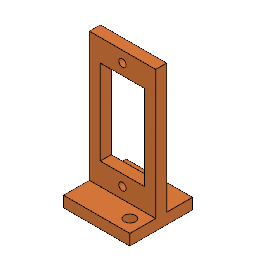
chassis laser 2x3mm (Autodesk Fusion 360 archive; units mm, degrees)
design "Version 3D vissée"
Autodesk Fusion 360 part; units mm, degrees
sketch "Sketch base" plane through (0, 0, 0) normal (0, 1, 0) x (1, 0, 0)
  line L0 (0, 0) -> (18, 0)
  line L1 (18, 0) -> (18, -3)
  line L2 (18, -3) -> (0, -3)
  line L3 (0, -3) -> (0, 0)
  dimension "d1" = 18
  dimension "d2" = 3
  constraint horizontal L0
  constraint vertical L1
  constraint horizontal L2
  constraint vertical L3
  constraint coincident L0.start L3.end
  measures "d1" distance of L0.start L0.end
  measures "d2" distance of L0.start L2.end
extrude "Extrude base" add sketch "Sketch base" along normal blind 38
sketch "Sketch face" plane through (0, 0, 0) normal (0, 0, -1) x (-1, 0, 0)
  line L0 (-18, 0) -> (0, 0)
  line L1 (0, 0) -> (0, 38)
  line L2 (0, 38) -> (-18, 38)
  line L3 (-18, 38) -> (-18, 0)
  circle A0 centre (-9, 35) radius 1
  circle A1 centre (-9, 6) radius 1
  line L4 (-15, 32) -> (-3, 32)
  line L5 (-3, 32) -> (-3, 9)
  line L6 (-3, 9) -> (-15, 9)
  line L7 (-15, 9) -> (-15, 32)
  line L8 (0, 0) -> (-18, 0)
  line L9 (-18, 0) -> (-18, 3)
  line L10 (-18, 3) -> (0, 3)
  line L11 (0, 3) -> (0, 0)
  dimension "d5" = 2
  dimension "d6" = 2
  dimension "d7" = 12
  dimension "d8" = 3
  dimension "d9" = 3
  dimension "d10" = 3
  dimension "d13" = 3
  dimension "d14" = 9
  dimension "d15" = 9
  dimension "d19" = 3
  dimension "d34" = 23
  constraint horizontal L4
  constraint vertical L5
  constraint horizontal L6
  constraint vertical L7
  constraint horizontal L8
  constraint vertical L9
  constraint horizontal L10
  constraint vertical L11
  constraint coincident L0.end L1.start
  measures "d5" diameter of A0
  measures "d6" diameter of A1
  measures "d7" distance of L4.start L4.end
  measures "d8" distance of L3 L7
  measures "d9" distance of A0.centre L4
  measures "d10" distance of A1.centre L6
  measures "d13" distance of L2 A0.centre
  measures "d14" distance of L1 A0.centre
  measures "d15" distance of L1 A1.centre
  measures "d19" distance of L0.end L10.end
  measures "d34" distance of L4 L6
extrude "Extrude face" cut sketch "Sketch face" against normal blind 4 contours A0 | A1 | L4 L5 L6 L7
extrude "Extrude socle" add sketch "Sketch face" along normal blind 7 and the other way blind 10 contours L0 L1 L3 L8 L9 L10 L11
hole "Hole1" at (3.5, 3, -3.5) direction (0, -1, 0) diameter 3 depth 5 tip angle 180
hole "Hole2" at (14.5, 3, 6.5) direction (0, -1, 0) diameter 3 depth 5 tip angle 180
named bodies: "Fixateur"

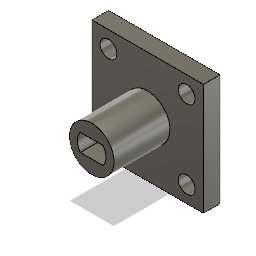
design "Fixation"
Autodesk Fusion 360 part; units mm, degrees
sketch "Sketch1" plane through (0, 0, 0) normal (0, 0, 1) x (1, 0, 0)
  line L0 (2.55, 1.55) -> (-2.55, -1.55) construction
  line L1 (2.55, 1.55) -> (-2.55, -1.55) construction
  line L2 (-2.55, 1.55) -> (-2.55, -1.55)
  circle A0 centre (0, 0) radius 4
  line L3 (-2.55, 1.55) -> (2.55, -1.55) construction
  line L4 (-2.55, -1.55) -> (2.55, -1.55)
  line L5 (2.55, 1.55) -> (-2.55, 1.55)
  line L6 (2.55, 1.55) -> (-2.55, -1.55) construction
  line L7 (-2.55, 1.55) -> (2.55, -1.55) construction
  line L8 (-2.55, 1.55) -> (2.55, -1.55) construction
  circle A1 centre (0, 0) radius 2.55
  line L9 (2.55, -1.55) -> (2.55, 1.55)
  line L10 (-10, 10) -> (10, 10)
  line L11 (10, 10) -> (10, -10)
  line L12 (10, -10) -> (-10, -10)
  line L13 (-10, -10) -> (-10, 10)
  circle A2 centre (-7, 7) radius 1.5
  line L14 (0, 10) -> (0, 7.5)
  circle A3 centre (7, 7) radius 1.5
  line L15 (-10, 0) -> (-8.5, 0)
  circle A4 centre (-7, -7) radius 1.5
  circle A5 centre (7, -7) radius 1.5
  dimension "d1" = 5.1
  dimension "d2" = 5.1
  dimension "d3" = 3.1
  dimension "d4" = 8
  dimension "d5" = 5.1
  dimension "d6" = 5.1
  dimension "d7" = 20
  dimension "d8" = 20
  dimension "d9" = 3
  measures "d4" diameter of A0
  measures "d5" diameter of A1
  measures "d9" diameter of A2
extrude "Extrude1" add sketch "Sketch1" along normal blind 10 contours L2 L5 A1 | L2 L4 A1 | L5 A1 | L4 A1 | L5 A1 L9 | L4 A1 L9 | A0 makes body 1
extrude "Extrude2" add sketch "Sketch1" against normal blind 3 separate body contours L10 L11 L12 L13 makes body 2
extrude "Extrude3" add sketch "Sketch1" against normal blind 3 contours L2 L5 A1 | L2 L4 A1 | L4 L5 A1 | L5 A1 | L4 A1 | L5 A1 L9 | L4 A1 L9 | A0 bodies 1 2

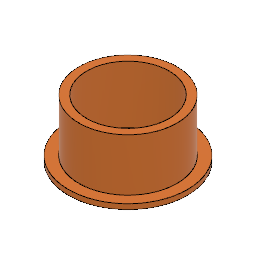
design "petit guide feutre 3d"
Autodesk Fusion 360 part; units mm, degrees
sketch "Sketch tranche" plane through (0, 0, 0) normal (0, 0, 1) x (1, 0, 0)
  line L0 (0, 0) -> (1.5, 0)
  line L1 (1.5, 0) -> (1.5, 11)
  line L2 (1.5, 11) -> (0, 11)
  line L3 (0, 11) -> (0, 0)
  line L4 (-7.875, 0) -> (-7.875, 6)
  line L5 (1.5, 0) -> (3.5, 0)
  line L6 (3.5, 0) -> (3.5, 1)
  line L7 (3.5, 1) -> (1.5, 1)
  line L8 (1.5, 1) -> (1.5, 0)
  dimension "d1" = 11
  dimension "d2" = 1.5
  dimension "d3" = 7.875
  dimension "d5" = 2
  dimension "d6" = 1
  constraint horizontal L0
  constraint vertical L1
  constraint horizontal L2
  constraint vertical L3
  constraint coincident L0.start L3.end
  constraint vertical L4
  constraint horizontal L5
  constraint vertical L6
  constraint horizontal L7
  constraint vertical L8
  measures "d1" distance of L0.start L2.end
  measures "d2" distance of L0.start L0.end
  measures "d3" distance of L3 L4
  measures "d5" distance of L0.end L5.end
  measures "d6" distance of L0.end L7.end
revolve "Revolution tranche" add sketch "Sketch tranche" angle 360 about axis through (-7.875, 0, 0) along (0, 1, 0)
revolve "Revolve1" [suppressed]
named bodies: "tube", "Guide feutre"

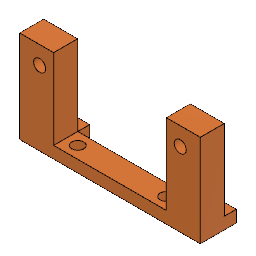
design "Fixateur double - 2D"
Autodesk Fusion 360 part; units mm, degrees
sketch "Sketch principal" plane through (0, 0, 0) normal (0, 0, 1) x (1, 0, 0)
  line L0 (45, 0) -> (45, 23)
  line L1 (45, 23) -> (36.5, 23)
  line L2 (36.5, 0) -> (45, 0)
  line L3 (36.5, 23) -> (36.5, 0)
  circle A0 centre (40, 18.5) radius 1.5
  line L4 (8.5, 23) -> (0, 23)
  line L5 (0, 0) -> (8.5, 0)
  line L6 (0, 23) -> (0, 0)
  line L7 (8.5, 0) -> (8.5, 23)
  circle A1 centre (5, 18.5) radius 1.5
  line L8 (8.5, 0) -> (36.5, 0)
  line L9 (36.5, 0) -> (36.5, 3)
  line L10 (36.5, 3) -> (8.5, 3)
  line L11 (8.5, 3) -> (8.5, 0)
  line L12 (8.5, 3) -> (0, 3)
  line L13 (0, 3) -> (0, 0)
  line L14 (0, 0) -> (8.5, 0)
  line L15 (8.5, 0) -> (8.5, 3)
  line L16 (36.5, 3) -> (45, 3)
  line L17 (45, 3) -> (45, 0)
  line L18 (45, 0) -> (36.5, 0)
  line L19 (36.5, 0) -> (36.5, 3)
  point P0 (36.5, 0)
  dimension "d15" = 23
  dimension "d16" = 8.5
  dimension "d17" = 3
  dimension "d18" = 4.5
  dimension "d20" = 23
  dimension "d21" = 8.5
  dimension "d22" = 3
  dimension "d23" = 4.5
  dimension "d24" = 3.5
  dimension "d25" = 28
  dimension "d26" = 3.5
  dimension "d28" = 3
  dimension "d29" = 28
  constraint horizontal L2
  constraint vertical L0
  constraint horizontal L1
  constraint vertical L3
  constraint coincident P0 L2.start
  constraint horizontal L5
  constraint vertical L7
  constraint horizontal L4
  constraint vertical L6
  constraint coincident L5.start L6.end
  constraint horizontal L8
  constraint vertical L9
  constraint horizontal L10
  constraint vertical L11
  constraint horizontal L12
  constraint vertical L13
  constraint horizontal L14
  constraint vertical L15
  constraint horizontal L16
  constraint vertical L17
  constraint horizontal L18
  constraint vertical L19
  measures "d15" distance of P0 L1.end
  measures "d16" distance of P0 L0.start
  measures "d17" diameter of A0
  measures "d18" distance of A0.centre L1
  measures "d20" distance of L5.start L4.end
  measures "d21" distance of L5.start L5.end
  measures "d22" diameter of A1
  measures "d23" distance of A1.centre L4
  measures "d24" distance of A1.centre L7
  measures "d25" distance of L3 L7
  measures "d26" distance of A0.centre L3
  measures "d28" distance of L5.end L10.end
  measures "d29" distance of L9.end L10.end
extrude "Extrude affichage" add sketch "Sketch principal" along normal blind 6
ref_plane "WorkPlane1" through (22.5, 13, 3) normal (1, 0, 0) x (0, 1, 0)
ref_plane "WorkPlane2" through (22.5, 11.5, 3) normal (0, 0, -1) x (-1, 0, 0)
sketch "Sketch4" plane through (0, 3, 0) normal (0, 1, 0) x (-1, 0, 0)
  line L0 (-36.5, 0) -> (-8.5, 0)
  line L1 (-8.5, 0) -> (-8.5, 6)
  line L2 (-8.5, 6) -> (-36.5, 6)
  line L3 (-36.5, 6) -> (-36.5, 0)
  circle A0 centre (-11.5, 3) radius 1.5
  line L4 (-22.5, 0) -> (-22.5, 6)
  circle A1 centre (-33.5, 3) radius 1.5
  dimension "d32" = 3
  dimension "d35" = 3
  constraint midpoint L0 L4.start
  constraint midpoint L2 L4.end
  constraint symmetric A0 L4 A1
  measures "d32" diameter of A0
  measures "d35" distance of L1 A0.centre
extrude "Extrude2" cut sketch "Sketch4" against normal blind 11 contours A0 | A1
extrude "Extrude3" add sketch "Sketch principal" against normal blind 3 contours L0 L2 L3 L9 L16 L17 L18 L19 | L5 L6 L7 L11 L12 L13 L14 L15
named bodies: "Fixateur U"

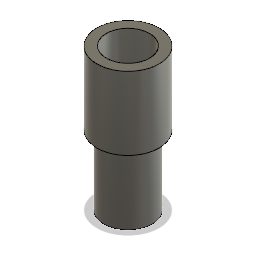
design "Guide feutre 3D"
Autodesk Fusion 360 part; units mm, degrees
sketch "Sketch tranche" plane through (0, 0, 0) normal (0, 0, 1) x (1, 0, 0)
  line L0 (0, 0) -> (0.8, 0)
  line L1 (0.8, 0) -> (0.8, 21)
  line L2 (0.8, 21) -> (0, 21)
  line L3 (0, 21) -> (0, 0)
  line L4 (-6.2, 0) -> (-6.2, 6)
  line L5 (0.8, 0) -> (2.8, 0)
  line L6 (2.8, 0) -> (2.8, 21)
  line L7 (2.8, 21) -> (0.8, 21)
  line L8 (0.8, 21) -> (0.8, 0)
  line L9 (0, 0) -> (0.8, 0)
  line L10 (0.8, 0) -> (0.8, -20)
  line L11 (0.8, -20) -> (0, -20)
  line L12 (0, -20) -> (0, 0)
  dimension "d1" = 21
  dimension "d2" = 0.8
  dimension "d3" = 6.2
  dimension "d5" = 2
  dimension "d6" = 21
  dimension "d8" = 20
  dimension "d9" = 0.8
  measures "d3" distance of L3 L4
  measures "d5" distance of L0.start
  measures "d8" distance of L0.start
revolve "Revolve3" add sketch "Sketch tranche" angle 360 about axis through (-6.2, 0, 0) along (0, 1, 0)

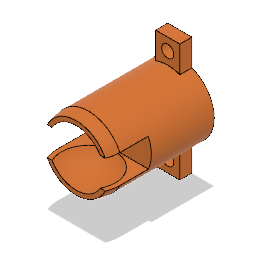
design "Fixateur bille - flexible"
Autodesk Fusion 360 part; units mm, degrees
sphere "Sphère de départ" add diameter 17 placed x (1, 0, 0) y (0, 0, -1) z (0, 1, 0) at (0, 0, 0) makes body 1
shell "Evidage sphère" thickness 1 removed faces 0 bodies 1
ref_plane "WorkPlane1" through (0, 0, 3) normal (0, 0, 1) x (1, 0, 0)
split "Section avant" by plane through (0, 0, 3) normal (0, 0, 1) bodies 1 makes body 2 at (-5.4981, 0.571, 6.4572)
delete_body "RemoveBody1" bodies 2
cylinder "Cylindre extension" add diameter 17 height -22.5 placed x (1, 0, 0) y (0, 1, 0) z (0, 0, 1) at (0, 0, 0) separate body makes body 3
sphere "Shère évidage cylindre" cut diameter 15 placed x (1, 0, 0) y (0, 0, -1) z (0, 1, 0) at (0, 0, 0) bodies 3
combine "Combine1" operation add target body 1 tool bodies 3
ref_plane "WorkPlane4" through (0, 8.5, -11.25) normal (0, 1, 0) x (1, 0, 0)
sketch "Sketch vis haut" plane through (0, 8.5, -4.25) normal (0, 1, 0) x (1, 0, 0)
  line L0 (0, 18.25) -> (0, 16.75)
  line L1 (-3, 18.25) -> (3, 18.25)
  line L2 (3, 18.25) -> (3, 15.25)
  line L3 (3, 15.25) -> (-3, 15.25)
  line L4 (-3, 15.25) -> (-3, 18.25)
  line L5 (0, 16.75) -> (0.1, 16.75)
  point P0 (0, 16.75)
  point P1 (0, 18.25)
  dimension "d72" = 1.5
  dimension "d73" = 3
  dimension "d74" = 6
  constraint coincident P1 L0.start
  constraint coincident P0 L0.end
  constraint vertical L0
  constraint horizontal L1
  constraint vertical L2
  constraint horizontal L3
  constraint vertical L4
  constraint symmetric L0 L2 L4
  constraint perpendicular L0 L5
  constraint symmetric L1 L3 L5
  measures "d72" distance of P0 L0.start
  measures "d73" distance of L1.end L2.end
  measures "d74" distance of L2 L4
extrude "Extrude vis haut" add sketch "Sketch vis haut" along normal blind 6 and the other way blind 2 separate body makes body 4
hole "Trou vis haut" at (0, 11.5, -19.5) direction (0, 0, -1) diameter 3 depth 3 tip angle 180 bodies 4
mirror "Mirroir vis" about plane through (0, 0, 0) normal (0, 1, 0) of bodies 4 makes body 5
combine "Combine2" operation add target body 1 tool bodies 4 5
sketch "Sketch13" plane through (0, 0, 3) normal (0, 0, 1) x (1, 0, 0)
  line L0 (9, 3.5) -> (-9, 3.5)
  line L1 (-9, 3.5) -> (-9, -3.5)
  line L2 (-9, -3.5) -> (9, -3.5)
  line L3 (9, -3.5) -> (9, 3.5)
  line L4 (9, 3.5) -> (-9, -3.5) construction
  line L5 (-9, 3.5) -> (9, -3.5) construction
  dimension "d54" = 7
  dimension "d55" = 18
  constraint perpendicular L0 L1
  constraint parallel L0 L2
  constraint parallel L1 L3
  constraint horizontal L0
  constraint coincident L4 origin
  constraint coincident L5 origin
  measures "d54" distance of L0.end L1.end
  measures "d55" distance of L1.end L2.end
extrude "Extrude écartement" cut sketch "Sketch13" against normal blind 10 bodies 1
named bodies: "Fixateur"
